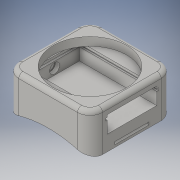
# Autodesk Inventor part: Track v3
Saved by Autodesk Inventor 2016 (Build 200138000, 138)
## iProperties
Created: 2016-05-24
Part Number: Track v3
Material: Generic
Document SubType Name: Modeling
Designer: xdlea
Density: 1 g/cm^3
Appearance: Default
Author: xdlea
Autodesk Inventor part; units mm, degrees
ref_plane "YZ Plane" through (0, 0, 0) normal (1, 0, 0) x (0, 1, 0)
ref_plane "XZ Plane" through (0, 0, 0) normal (0, 1, 0) x (-1, 0, 0)
ref_plane "XY Plane" through (0, 0, 0) normal (0, 0, 1) x (1, 0, 0)
sketch "Sketch1" plane through (0, 0, 0) normal (0, 0, 1) x (1, 0, 0)
  arc A0 (31.877, -6.35) -> (-31.877, -6.35) centre (0, -83.1863) ccw
  line L0 (-31.877, -6.35) -> (31.877, -6.35) construction
  line L1 (0, 36.3731) -> (0, -103.1128) construction
  line L2 (-44.6278, 0) -> (44.6278, 0) construction
  line L3 (-31.877, -6.35) -> (-31.877, -4.497)
  line L4 (-31.877, 16.4465) -> (31.877, 16.4465)
  line L5 (31.877, 16.4465) -> (31.877, -2.4453)
  line L6 (-30.1625, 16.4465) -> (-30.1625, 5.334) construction
  line L7 (-30.1625, 5.334) -> (30.1625, 5.334) construction
  line L8 (30.1625, 5.334) -> (30.1625, 16.4465) construction
  arc A1 (31.877, -4.497) -> (-31.877, -4.497) centre (0, -83.1863) ccw
  arc A2 (31.877, -2.4453) -> (-31.877, -2.4453) centre (0, -83.1863) ccw
  line L9 (-30.1625, 13.1134) -> (-26.9875, 13.1134) construction
  line L10 (-26.9875, 13.1134) -> (-26.9875, 5.334) construction
  line L11 (30.1625, 12.4907) -> (26.9875, 12.4907) construction
  line L12 (26.9875, 12.4907) -> (26.9875, 5.334) construction
  line L13 (-31.877, -2.4453) -> (-31.877, 16.4465)
  line L14 (-31.877, -4.497) -> (-31.877, -2.4453)
  line L15 (31.877, -2.4453) -> (31.877, -4.497)
  line L16 (31.877, -4.497) -> (31.877, -6.35)
  point P0 (0, 0)
  point P1 (0, 3.6195)
  dimension "d0" = 1.7145
  dimension "d2" = 1.7145
  dimension "d3" = 1.905
  dimension "d4" = 1.7145
  dimension "d5" = 1.7145
  dimension "d6" = 11.1125
  dimension "d7" = 3.175
  dimension "d8" = 3.175
  dimension "d10" = 60.325
  dimension "d11" = 6.35
  constraints: 30 end point, 10 parallel, 9 perpendicular, 8 point on circle, 7 point on line, 4 vertical, 3 centre point, 2 concentric, 1 symmetric about line
  measures "d0" distance between parallel lines of L3 L6
  measures "d2" distance between parallel lines of L5 L8
  measures "d3" radial gap between concentric circles of A1 A2
  measures "d4" radial gap between concentric circles of A0 A1
  measures "d5" distance from line of point (0, 3.62) L7
  measures "d6" distance of L7.end L8.end
  measures "d7" distance between parallel lines of L10 L6
  measures "d8" distance between parallel lines of L8 L12
  measures "d10" distance between parallel lines of L8 L6
  measures "d11" vertical distance of point (0, 0) L0.end
extrude "Extrusion1" add sketch "Sketch1" along normal mid plane 63.754
sketch "Sketch2" plane through (-31.877, 16.4465, 31.877) normal (0, 1, 0) x (1, 0, 0)
  line L0 (62.0395, 1.7145) -> (1.7145, 1.7145)
  line L1 (1.7145, 1.7145) -> (1.7145, 11.684)
  line L2 (1.7145, 62.0395) -> (62.0395, 62.0395)
  line L3 (62.0395, 62.0395) -> (62.0395, 52.07)
  line L4 (62.0395, 1.7145) -> (1.7145, 62.0395) construction
  line L5 (1.7145, 1.7145) -> (62.0395, 62.0395) construction
  line L6 (0, 63.754) -> (0, 0) projected
  line L7 (76.5048, 31.877) -> (-12.7508, 31.877) construction
  line L8 (31.877, 76.5048) -> (31.877, -12.7508) construction
  line L9 (1.7145, 11.684) -> (62.0395, 11.684)
  line L10 (1.7145, 11.684) -> (1.7145, 52.07)
  line L11 (1.7145, 52.07) -> (62.0395, 52.07)
  line L12 (1.7145, 52.07) -> (1.7145, 62.0395)
  line L13 (62.0395, 11.684) -> (62.0395, 1.7145)
  line L14 (0, 63.754) -> (63.754, 63.754) projected
  line L15 (4.8895, 50.8) -> (63.754, 50.8)
  line L16 (4.8895, 50.8) -> (4.8895, 12.954)
  line L17 (63.754, 63.754) -> (63.754, 0) projected
  line L18 (63.754, 50.8) -> (63.754, 12.954)
  line L19 (63.754, 0) -> (63.754, 63.754) projected
  line L20 (4.8895, 12.954) -> (63.754, 12.954)
  line L21 (62.0395, 11.684) -> (63.754, 11.684)
  line L22 (63.754, 12.954) -> (63.754, 11.684)
  line L23 (62.0395, 52.07) -> (63.754, 52.07)
  line L24 (63.754, 52.07) -> (63.754, 50.8)
  point P0 (31.877, 31.877)
  dimension "d14" = 1.7145
  dimension "d17" = 1.7145
  dimension "d34" = 1.27
  dimension "d35" = 1.7145
  dimension "d36" = 3.175
  dimension "d37" = 40.386
  constraints: 38 end point, 12 perpendicular, 7 parallel, 5 point on line, 2 midpoint, 1 horizontal, 1 vertical, 2 other
  measures "d14" distance between parallel lines of L6 L1
  measures "d17" distance between parallel lines of L14 L2
  measures "d34" distance between parallel lines of L15 L11
  measures "d35" distance between parallel lines of L17 L3
  measures "d36" distance between parallel lines of L10 L16
  measures "d37" distance of L1.end L10.end
extrude "Extrusion2" cut sketch "Sketch2" against normal blind 11.1125 contours L20 L16 L15 L17
extrude "Extrusion3" cut sketch "Sketch2" against normal blind 1.778 contours L9 L10 L11 L23 L17 L15 L16 L20 L21
extrude "Extrusion6" cut sketch "Sketch1" along normal mid plane 26.035 contours A1 L14 A2 L15
fillet "Fillet1" radius 9.525 4 edges at (31.877, 5.0483, 31.877) (31.877, 5.0483, -31.877) (-31.877, 5.0483, 31.877) (-31.877, 5.0483, -31.877)
sketch "Sketch6" plane through (-26.9875, 5.334, 18.923) normal (1, 0, 0) x (0, 0, -1)
  circle A0 centre (18.923, 4.6673) radius 3.81
  circle A1 centre (18.923, 4.6673) radius 2.8575
  line L0 (0, 0) -> (0, 9.3345) projected
  line L1 (37.846, 0) -> (0, 0) projected
  point P0 (18.923, -5.334)
  point P1 (0, 4.6673)
  point P2 (18.923, 0)
  dimension "d38" = 7.62
  dimension "d39" = 5.715
  constraints: 2 centre point, 2 midpoint, 1 coincident, 1 horizontal alignment, 1 vertical alignment
  measures "d38" diameter of A0
  measures "d39" diameter of A1
extrude "Extrusion7" cut sketch "Sketch6" against normal up to next contours A1
extrude "Extrusion8" cut sketch "Sketch6" against normal blind 3.175
sketch "Sketch7" plane through (-30.1625, 16.4465, 20.193) normal (0, 1, 0) x (1, 0, 0)
  line L0 (7.8105, 52.07) -> (52.5145, 52.07) projected
  arc A0 (7.8105, 52.07) -> (-1.7145, 42.545) centre (7.8105, 42.545) ccw projected
  arc A1 (62.0395, 42.545) -> (52.5145, 52.07) centre (52.5145, 42.545) ccw projected
  line L1 (-1.7145, -2.159) -> (-1.7145, 42.545) projected
  arc A2 (-1.7145, -2.159) -> (7.8105, -11.684) centre (7.8105, -2.159) ccw projected
  line L2 (52.5145, -11.684) -> (7.8105, -11.684) projected
  arc A3 (52.5145, -11.684) -> (62.0395, -2.159) centre (52.5145, -2.159) ccw projected
  line L3 (62.0395, 42.545) -> (62.0395, 40.386) projected
  line L4 (62.0395, 42.545) -> (62.0395, 39.116)
  line L5 (62.0395, 39.116) -> (3.175, 39.116) projected
  line L6 (3.175, 39.116) -> (3.175, 1.27) projected
  line L7 (3.175, 1.27) -> (62.0395, 1.27) projected
  line L8 (62.0395, 39.116) -> (62.0395, 1.27)
  line L9 (62.0395, 1.27) -> (62.0395, -2.159)
  point P0 (30.1625, 20.193)
  constraints: 8 end point, 3 vertical
extrude "Extrusion9" add sketch "Sketch7" along normal blind 1.778 contours L0 A1 L3 L4 L5 L6 L7 L9 A3 L2 A2 L1 A0
sketch "Sketch8" plane through (-30.1625, 18.2245, 20.193) normal (0, 1, 0) x (1, 0, 0)
  line L0 (52.5145, 52.07) -> (7.8105, 52.07) projected
  arc A0 (62.0395, 42.545) -> (52.5145, 52.07) centre (52.5145, 42.545) ccw projected
  arc A1 (7.8105, 52.07) -> (-1.7145, 42.545) centre (7.8105, 42.545) ccw projected
  line L1 (-1.7145, 42.545) -> (-1.7145, -2.159) projected
  arc A2 (-1.7145, -2.159) -> (7.8105, -11.684) centre (7.8105, -2.159) ccw projected
  line L2 (7.8105, -11.684) -> (52.5145, -11.684) projected
  arc A3 (52.5145, -11.684) -> (62.0395, -2.159) centre (52.5145, -2.159) ccw projected
  line L3 (62.0395, -2.159) -> (62.0395, 42.545) projected
  line L4 (62.0395, 42.545) -> (62.0395, -2.159)
  circle A4 centre (30.1625, 20.193) radius 27.94
  dimension "d47" = 55.88
  constraints: 2 end point, 1 centre point, 1 coincident, 1 collinear, 1 tangent
  measures "d47" diameter of A4
extrude "Extrusion10" add sketch "Sketch8" along normal blind 6.35
fillet "Fillet2" radius 3.175 8 edges at (29.0872, 24.5745, 29.0872) (31.877, 24.5745, 0) (29.0872, 24.5745, -29.0872) (0, 24.5745, -31.877) (-29.0872, 24.5745, -29.0872) (-31.877, 24.5745, 0) (-29.0872, 24.5745, 29.0872) (0, 24.5745, 31.877)
equation "\"d17\" = d14"
equation "\"d35\" = d17"
equation "\"d18\" = d6"
body "Solid1"
